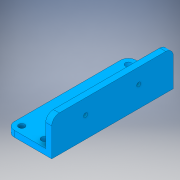
# Autodesk Inventor part: Realsense
Saved by Autodesk Inventor 2019 (Build 230136000, 136)
## iProperties
Created: 2019-12-14
Part Number: Realsense
Material: Generic
Document SubType Name: Modeling
Designer: james
Density: 1 g/cm^3
Appearance: Default(1)
Author: james
Autodesk Inventor part; units mm, degrees
ref_plane "YZ Plane" through (0, 0, 0) normal (1, 0, 0) x (0, 1, 0)
ref_plane "XZ Plane" through (0, 0, 0) normal (0, 1, 0) x (-1, 0, 0)
ref_plane "XY Plane" through (0, 0, 0) normal (0, 0, 1) x (1, 0, 0)
sketch "Sketch1" plane through (0, 0, 0) normal (1, 0, 0) x (0, 1, 0)
  line L0 (6.3049, 39.363) -> (-19.0951, 39.363)
  line L1 (-19.0951, 39.363) -> (-19.0951, -63.507)
  line L2 (-19.0951, -63.507) -> (6.3049, -63.507)
  line L3 (6.3049, -63.507) -> (6.3049, 39.363)
  point P0 (0, 0)
  dimension "d0" = 102.87
  dimension "d1" = 25.4
  constraints: 8 end point, 2 parallel, 1 horizontal, 1 perpendicular
  measures "d0" distance of L0.end L1.end
  measures "d1" distance of L0.start L0.end
extrude "Extrusion1" add sketch "Sketch1" along normal blind 5.08
fillet "Fillet1" radius 6.35 2 edges at (2.54, 6.3049, 39.363) (2.54, 6.3049, -63.507)
sketch "Sketch7" plane through (0, -19.0951, 39.363) normal (0, 0, 1) x (1, 0, 0)
  line L0 (0, 0) -> (5.08, 0)
  line L1 (5.08, 0) -> (5.08, -5.08)
  line L2 (5.08, -5.08) -> (-33.02, -5.08)
  line L3 (-33.02, -5.08) -> (-33.02, 0)
  line L4 (-33.02, 0) -> (0, 0)
  line L5 (0, 0) -> (0, 0)
  line L6 (0, 0) -> (5.08, 0) projected
  line L7 (0, 19.05) -> (0, 0) projected
  point P0 (0, 19.0951)
  dimension "d51" = 5.08
  dimension "d52" = 5.08
  dimension "d53" = 90
  dimension "d54" = 5.08
  dimension "d55" = 38.1
  dimension "d56" = 0
  dimension "d57" = 0
  constraints: 12 end point, 3 perpendicular, 1 horizontal, 1 parallel
  measures "d51" distance of L0.start L0.end
  measures "d52" distance of L0.end L1.end
  measures "d53" angle of L2 L1
  measures "d54" distance of L2.end L3.end
  measures "d55" distance of L1.end L2.end
  measures "d56" distance between parallel lines of L0 L6
  measures "d57" distance between parallel lines of L7 L5
extrude "Extrusion4" add sketch "Sketch7" against normal blind 102.87
fillet "Fillet2" radius 6.35 2 edges at (-33.02, -21.6351, -63.507) (-33.02, -21.6351, 39.363)
sketch "Sketch15" plane through (5.08, 0, 0) normal (1, 0, 0) x (0, 0, -1)
  line L0 (-39.363, -0.0451) -> (-39.363, -24.1751) projected
  line L1 (63.507, -0.0451) -> (63.507, -24.1751) projected
  line L2 (57.157, 6.3049) -> (-33.013, 6.3049) projected
  point P0 (0, 0)
  point P1 (-10.788, -6.3951)
  point P2 (34.2208, -6.3951)
  dimension "d143" = 0
  dimension "d144" = 45.0088
  dimension "d145" = 28.575
  dimension "d146" = 29.2862
  dimension "d147" = 12.7
  measures "d143" vertical distance of point (34.221, -6.395) point (-10.788, -6.395)
  measures "d144" distance of point (-10.788, -6.395) point (34.221, -6.395)
  measures "d145" distance from line of L0 point (-10.788, -6.395)
  measures "d146" distance from line of L1 point (34.221, -6.395)
  measures "d147" distance from line of L2 point (-10.788, -6.395)
hole "Hole7" at (5.08, -6.3951, 10.788) at (5.08, -6.3951, -34.2208) direction (-1, 0, 0) diameter 3.4036 depth 25.4 tip angle 118 clearance for "Flat Head Machine Screw" size "M3" standard "Ansi Metric M Profile"
sketch "Sketch16" plane through (5.08, -24.1751, -63.507) normal (0, -1, 0) x (1, 0, 0)
  line L0 (0, 102.87) -> (0, 0) projected
  line L1 (0, 102.87) -> (-31.75, 102.87) projected
  line L2 (-38.1, 96.52) -> (-38.1, 6.35) projected
  line L3 (0, 0) -> (-31.75, 0) projected
  point P0 (-5.08, 63.507)
  point P1 (-12.7, 96.52)
  point P2 (-31.75, 96.52)
  point P3 (-31.75, 6.35)
  point P4 (-12.7, 6.35)
  dimension "d155" = 0
  dimension "d156" = 0
  dimension "d157" = 0
  dimension "d158" = 0
  dimension "d159" = 12.7
  dimension "d160" = 6.35
  dimension "d161" = 6.35
  dimension "d162" = 6.35
  measures "d155" horizontal distance of point (-12.7, 6.35) point (-12.7, 96.52)
  measures "d156" horizontal distance of point (-31.75, 96.52) point (-31.75, 6.35)
  measures "d157" vertical distance of point (-31.75, 6.35) point (-12.7, 6.35)
  measures "d158" vertical distance of point (-31.75, 96.52) point (-12.7, 96.52)
  measures "d159" distance from line of L0 point (-12.7, 96.52)
  measures "d160" distance from line of L1 point (-12.7, 96.52)
  measures "d161" distance from line of L2 point (-31.75, 96.52)
  measures "d162" distance from line of L3 point (-12.7, 6.35)
hole "Hole8" at (-7.62, -24.1751, 33.013) at (-26.67, -24.1751, 33.013) at (-26.67, -24.1751, -57.157) at (-7.62, -24.1751, -57.157) direction (0, 1, 0) diameter 5.1054 depth 25.4 tip angle 118 clearance for "Flat Head Machine Screw (82)" size "#10" standard "Ansi Unified Screw Threads"
body "Solid1"
